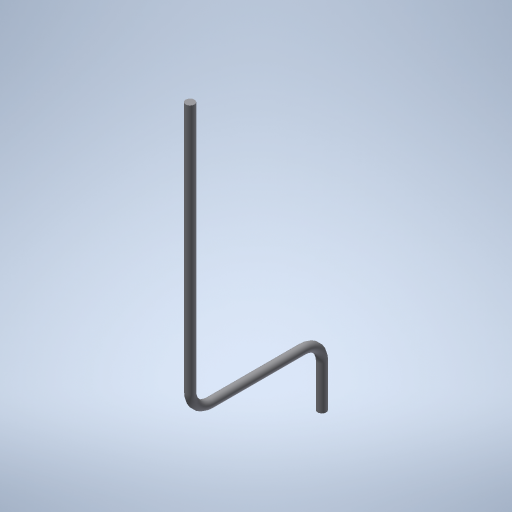
# Autodesk Inventor part: cable 2
Saved by Autodesk Inventor 2023 (Build 270158000, 158)
## iProperties
Created: 2022-10-17
Part Number: cable 2
Material: Generic
Document SubType Name: Modeling
Designer: Xiaba
Density: 1 g/cm^3
Appearance: Default
Author: Xiaba
Autodesk Inventor part; units mm, degrees
ref_plane "YZ Plane" through (0, 0, 0) normal (1, 0, 0) x (0, 1, 0)
ref_plane "XZ Plane" through (0, 0, 0) normal (0, 1, 0) x (-1, 0, 0)
sketch "Sketch1" plane through (0, 0, 0) normal (1, 0, 0) x (0, 1, 0)
  line L0 (67.821, 0) -> (56.1452, -2.7707)
  line L1 (67.821, 0) -> (0, 0)
  dimension "d2" = 12
  dimension "d10" = 67.821
  constraints: 4 end point, 1 horizontal
  measures "d2" distance of L0.start L0.end
  measures "d10" distance of L0.start L1.end
ref_plane "Work Plane1" through (0, 0, 0) normal (-1, 0, 0) x (0, 0, 1)
sketch "Sketch2" plane through (0, 0, 0) normal (-1, 0, 0) x (0, 0, 1)
  line L0 (0, 67.821) -> (0, 83.821)
  line L1 (-13.5147, 54.1452) -> (-13.5147, 49.7452)
  arc A0 (-11.5147, 56.1452) -> (-13.5147, 54.1452) centre (-11.5147, 54.1452) ccw
  line L2 (0, 67.821) -> (0, 58.1452)
  arc A1 (-2, 56.1452) -> (0, 58.1452) centre (-2, 58.1452) ccw
  line L3 (-2, 56.1452) -> (-11.5147, 56.1452)
  point P0 (-13.5147, 56.1452)
  dimension "d5" = 16
  dimension "d12" = 6.4
  dimension "d13" = 2
  dimension "d16" = 2
  constraints: 8 end point, 4 point on circle, 3 vertical, 2 centre point, 2 tangent, 1 horizontal, 1 point on line
  measures "d5" distance of L0.start L0.end
  measures "d12" distance of point (-13.515, 56.145) L1.end
  measures "d13" radius of A0
  measures "d16" radius of A1
ref_plane "Work Plane2" through (0, 83.821, 0) normal (0, 1, 0) x (-1, 0, 0)
sketch "Sketch3" plane through (0, 83.821, 0) normal (0, 1, 0) x (-1, 0, 0)
  circle A0 centre (0, 0) radius 0.45
  dimension "d6" = 0.9
  constraints: 1 centre point, 1 coincident
  measures "d6" diameter of A0
sweep "Sweep3" add profiles "Sketch3" path "Sketch2"
body "Solid4"
